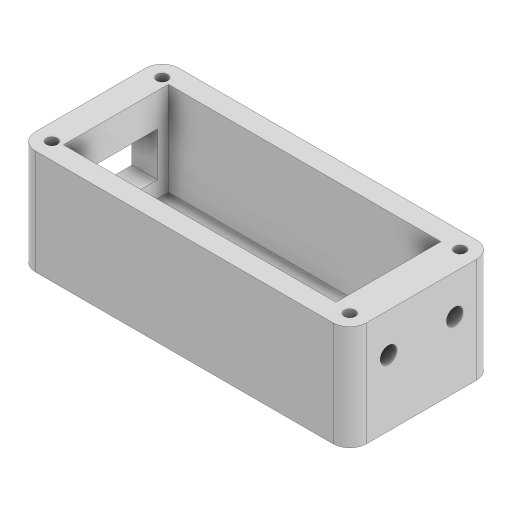
# Autodesk Inventor part: bawah
Saved by Autodesk Inventor 2023 (Build 270158000, 158)
## iProperties
Created: 2025-11-27
Part Number: bawah
Material: Generic
Document SubType Name: Modeling
Designer: dinoo
Density: 1 g/cm^3
Appearance: Default
Author: dinoo
Autodesk Inventor part; units mm, degrees
ref_plane "YZ Plane" through (0, 0, 0) normal (1, 0, 0) x (0, 1, 0)
ref_plane "XZ Plane" through (0, 0, 0) normal (0, 1, 0) x (-1, 0, 0)
ref_plane "XY Plane" through (0, 0, 0) normal (0, 0, 1) x (1, 0, 0)
sketch "Sketch1" plane through (0, 0, 0) normal (0, 1, 0) x (-1, 0, 0)
  line L0 (0, 0) -> (-60, 0)
  line L1 (-60, 0) -> (-60, -26)
  line L2 (-60, -26) -> (0, -26)
  line L3 (0, -26) -> (0, 0)
  line L4 (-54, -3.5) -> (-6, -3.5)
  line L5 (-6, -3.5) -> (-6, -22.5)
  line L6 (-6, -22.5) -> (-54, -22.5)
  line L7 (-54, -22.5) -> (-54, -3.5)
  line L8 (-54, -3.5) -> (-6, -22.5) construction
  line L9 (-6, -3.5) -> (-54, -22.5) construction
  point P0 (-30, -13)
  dimension "d0" = 60
  dimension "d2" = 48
  dimension "d3" = 6
  dimension "d4" = 6
  dimension "d36" = 19
  dimension "d37" = 3.5
  dimension "d38" = 3.5
  dimension "d39" = 26
  constraints: 20 end point, 4 parallel, 2 horizontal, 2 midpoint, 2 perpendicular
  measures "d0" distance of L2.end L1.end
  measures "d2" distance of L5.end L6.end
  measures "d3" distance between parallel lines of L3 L5
  measures "d4" distance between parallel lines of L1 L7
  measures "d36" distance between parallel lines of L6 L4
  measures "d37" distance between parallel lines of L0 L4
  measures "d38" distance between parallel lines of L2 L6
  measures "d39" distance between parallel lines of L2 L0
extrude "Extrusion1" add sketch "Sketch1" along normal blind 2 contours L3 L2 L1 L0 | L4 L5 L6 L7
extrude "Extrusion2" add sketch "Sketch1" along normal blind 19
sketch "Sketch2" plane through (0, 2, 0) normal (0, 1, 0) x (1, 0, 0)
  line L0 (6, 3.5) -> (54, 3.5) projected
  line L1 (54, 22.5) -> (6, 22.5) projected
  line L2 (54, 3.5) -> (48, 3.5)
  line L3 (48, 3.5) -> (48, 22.5)
  line L4 (48, 22.5) -> (54, 22.5)
  line L5 (54, 22.5) -> (54, 3.5)
  line L6 (6, 3.5) -> (6, 22.5) projected
  point P0 (0, 0)
  point P1 (48, 3.5)
  dimension "d11" = 42
  constraints: 8 end point, 2 parallel, 1 horizontal, 1 perpendicular, 1 point on line
  measures "d11" distance between parallel lines of L3 L6
extrude "Extrusion3" add sketch "Sketch2" along normal blind 3 contours L3 L1 L5 L0
sketch "Sketch3" plane through (0, 0, -3) normal (1, 0, 0) x (0, 0, -1)
  line L0 (-3, 0) -> (23, 0) projected
  line L1 (23, 0) -> (23, 19) projected
  line L2 (-3, 19) -> (23, 19) projected
  line L3 (-3, 0) -> (-3, 19) projected
  line L4 (2.5, 13) -> (17.5, 13)
  line L5 (17.5, 13) -> (17.5, 5)
  line L6 (17.5, 5) -> (2.5, 5)
  line L7 (2.5, 5) -> (2.5, 13)
  line L8 (2.5, 13) -> (17.5, 5) construction
  line L9 (17.5, 13) -> (2.5, 5) construction
  point P0 (-3, 0)
  point P1 (10, 9)
  point P2 (23, 9.5)
  point P3 (-3, 9.5)
  dimension "d14" = 5
  dimension "d15" = 8
  dimension "d16" = 5.5
  dimension "d17" = 5.5
  dimension "d18" = 15
  constraints: 12 end point, 4 midpoint, 2 parallel, 1 horizontal, 1 perpendicular
  measures "d14" distance between parallel lines of L0 L6
  measures "d15" distance of L4.end L5.end
  measures "d16" distance from line of point (23, 9.5) L5
  measures "d17" distance from line of point (-3, 9.5) L7
  measures "d18" distance of L4.start L4.end
extrude "Extrusion4" cut sketch "Sketch3" along normal blind 7.5 contours L4 L5 L6 L7
sketch "Sketch4" plane through (60, 0, 0) normal (1, 0, 0) x (0, 0, -1)
  circle A0 centre (7, 12) radius 1.5
  circle A1 centre (19, 12) radius 1.5
  line L0 (0, 0) -> (26, 0) projected
  line L1 (0, 0) -> (0, 19) projected
  line L2 (26, 0) -> (26, 19) projected
  dimension "d21" = 3
  dimension "d22" = 3
  dimension "d25" = 12
  dimension "d26" = 12
  dimension "d27" = 7
  dimension "d28" = 7
  constraints: 2 centre point
  measures "d21" diameter of A0
  measures "d22" diameter of A1
  measures "d25" distance from line of L0 A0.centre
  measures "d26" distance from line of L0 A1.centre
  measures "d27" distance from line of L1 A0.centre
  measures "d28" distance from line of L2 A1.centre
extrude "Extrusion5" cut sketch "Sketch4" against normal blind 7.5
fillet "Fillet1" radius 3 4 edges at (0, 9.5, 0) (0, 9.5, -26) (60, 9.5, 0) (60, 9.5, -26)
sketch "Sketch5" plane through (0, 19, 0) normal (0, 1, 0) x (1, 0, 0)
  arc A0 (60, 23) -> (57, 26) centre (57, 23) ccw projected
  line L0 (57, 26) -> (3, 26) projected
  arc A1 (3, 26) -> (0, 23) centre (3, 23) ccw projected
  line L1 (0, 23) -> (0, 3) projected
  arc A2 (0, 3) -> (3, 0) centre (3, 3) ccw projected
  line L2 (3, 0) -> (57, 0) projected
  arc A3 (57, 0) -> (60, 3) centre (57, 3) ccw projected
  line L3 (60, 3) -> (60, 23) projected
  line L4 (54, 3.5) -> (6, 3.5) projected
  line L5 (6, 3.5) -> (6, 22.5) projected
  line L6 (6, 22.5) -> (54, 22.5) projected
  line L7 (54, 22.5) -> (54, 3.5) projected
  circle A4 centre (3, 3) radius 1
  circle A5 centre (3, 23) radius 1
  circle A6 centre (57, 3) radius 1
  circle A7 centre (57, 23) radius 1
  point P0 (0, 0)
  dimension "d30" = 2
  dimension "d31" = 2
  dimension "d32" = 2
  dimension "d33" = 2
  constraints: 4 centre point, 4 coincident
  measures "d30" diameter of A4
  measures "d31" diameter of A5
  measures "d32" diameter of A6
  measures "d33" diameter of A7
extrude "Extrusion6" cut sketch "Sketch5" against normal blind 3 contours A4 | A5 | A6 | A7
sketch "Sketch6" plane through (0, 19, 0) normal (0, 1, 0) x (1, 0, 0)
  circle A0 centre (57, 3) radius 1 projected
  circle A1 centre (3, 23) radius 1 projected
  circle A2 centre (57, 23) radius 1 projected
  circle A3 centre (3, 3) radius 1 projected
  arc A4 (60, 23) -> (57, 26) centre (57, 23) ccw projected
  line L0 (57, 26) -> (3, 26) projected
  arc A5 (3, 26) -> (0, 23) centre (3, 23) ccw projected
  line L1 (0, 23) -> (0, 3) projected
  arc A6 (0, 3) -> (3, 0) centre (3, 3) ccw projected
  line L2 (3, 0) -> (57, 0) projected
  arc A7 (57, 0) -> (60, 3) centre (57, 3) ccw projected
  line L3 (60, 3) -> (60, 23) projected
  line L4 (54, 3.5) -> (6, 3.5) projected
  line L5 (6, 3.5) -> (6, 22.5) projected
  line L6 (6, 22.5) -> (54, 22.5) projected
  line L7 (54, 22.5) -> (54, 3.5) projected
  line L8 (6, 22.5) -> (6, 3.5) projected
  line L9 (6, 3.5) -> (4.6176, 3.5)
  line L10 (4.6176, 3.5) -> (4.6176, 22.5)
  line L11 (4.6176, 22.5) -> (6, 22.5)
  line L12 (6, 22.5) -> (6, 3.5)
  point P0 (0, 0)
  constraints: 8 end point, 2 parallel, 1 horizontal, 1 perpendicular
extrude "Extrusion7" cut sketch "Sketch6" against normal blind 17 contours L9 L10 L11 L5
equation "\"d38\" = d37"
equation "\"d17\" = d16"
equation "\"d26\" = d25"
equation "\"d28\" = d27"
body "Solid1"
